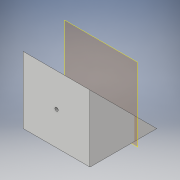
# Autodesk Inventor part: spiegelhalter
Saved by Autodesk Inventor 2017 (Build 210142000, 142)
## iProperties
Part Number: spiegelhalter
Material: Generisch
Document SubType Name: Modeling
Designer: Fabio
Density: 1 g/cm^3
Appearance: Vorgabe
Author: Fabio
Autodesk Inventor part; units mm, degrees
ref_plane "YZ Plane" through (0, 0, 0) normal (1, 0, 0) x (0, 1, 0)
ref_plane "XZ Plane" through (0, 0, 0) normal (0, 1, 0) x (-1, 0, 0)
ref_plane "XY Plane" through (0, 0, 0) normal (0, 0, 1) x (1, 0, 0)
sketch "Skizze1" plane through (0, 0, 0) normal (1, 0, 0) x (0, 1, 0)
  line L0 (0, 0) -> (0, -60)
  line L1 (0, -60) -> (60, -60)
  line L2 (60, -60) -> (0, 0)
  dimension "d0" = 45
  dimension "d1" = 60
  constraints: 6 end point, 1 perpendicular, 1 vertical
  measures "d0" angle of L0 L2
  measures "d1" distance of L0.end L1.end
extrude "Extrusion1" add sketch "Skizze1" along normal blind 60
ref_plane "Arbeitsebene1" through (0, 40, -60) normal (0, -1, 0) x (1, 0, 0)
sketch "Skizze3" plane through (0, 40, -60) normal (0, -1, 0) x (1, 0, 0)
  line L0 (0, 60) -> (60, 60) projected
  line L1 (0, 0) -> (0, 60) projected
  point P0 (30, 30)
  dimension "d7" = 30
  dimension "d8" = 30
  measures "d7" distance from line of L0 point (30, 30)
  measures "d8" distance from line of L1 point (30, 30)
hole "Bohrung1" at (30, 40, -30) direction (0, -1, 0) diameter 3 end through all counterbore diameter 10 counterbore depth 25
